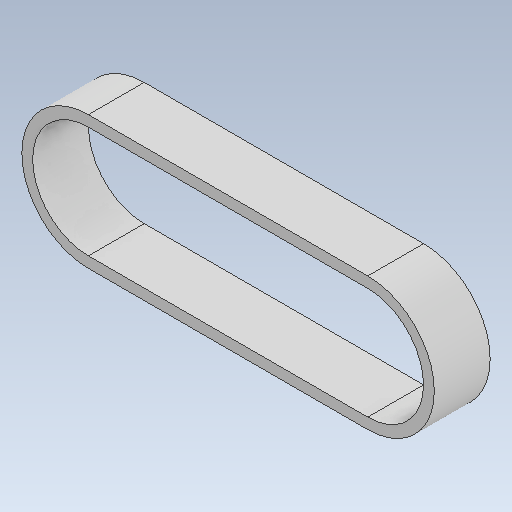
# Autodesk Inventor part: 43T timing belt from gobuilda
Saved by Autodesk Inventor 2020.2 (Build 242310000, 310)
## iProperties
Created: 2020-03-01
Part Number: 43T timing belt from gobuilda
Material: Generic
Document SubType Name: Modeling
Designer: deli
Density: 1 g/cm^3
Appearance: Default
Author: deli
Autodesk Inventor part; units mm, degrees
ref_plane "YZ Plane" through (0, 0, 0) normal (1, 0, 0) x (0, 1, 0)
ref_plane "XZ Plane" through (0, 0, 0) normal (0, 1, 0) x (-1, 0, 0)
ref_plane "XY Plane" through (0, 0, 0) normal (0, 0, 1) x (1, 0, 0)
sketch "Sketch1" plane through (0, 0, 0) normal (0, 0, 1) x (1, 0, 0)
  arc A0 (-67.0749, 30.1938) -> (-67.0749, 12.236) centre (-67.0749, 21.2149) ccw
  arc A1 (-22.075, 12.236) -> (-22.075, 30.1938) centre (-22.075, 21.2149) ccw
  line L0 (-67.0749, 30.1938) -> (-22.075, 30.1938)
  line L1 (-22.075, 12.236) -> (-67.0749, 12.236)
  line L2 (-22.075, 31.9338) -> (-67.0749, 31.9338)
  arc A2 (-67.0749, 31.9338) -> (-67.0749, 10.496) centre (-67.0749, 21.2149) ccw
  line L3 (-67.0749, 10.496) -> (-22.075, 10.496)
  arc A3 (-22.075, 10.496) -> (-22.075, 31.9338) centre (-22.075, 21.2149) ccw
  point P0 (0, 0)
  dimension "d0" = 17.9578
  dimension "d1" = 17.9578
  dimension "d2" = 0
  dimension "d3" = 44.9999
  dimension "d4" = 1.74
  constraints: 8 end point, 8 point on circle, 4 centre point, 2 tangent, 3 other
  measures "d0" diameter of A0
  measures "d1" diameter of A1
  measures "d2" vertical distance of A1.centre A0.centre
  measures "d3" distance of A1.centre A0.centre
  measures "d4" distance between parallel lines of L0 L2
extrude "Extrusion1" add sketch "Sketch1" along normal blind 9
body "Solid1"
